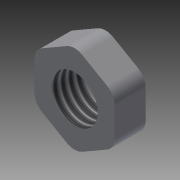
# Autodesk Inventor part: gaika3-2
Saved by Autodesk Inventor 2015 (Build 190159000, 159)
## iProperties
Created: 2016-05-20
Part Number: gaika3-2
Material: Generic
Document SubType Name: Modeling
Designer: Kostya
Density: 1 g/cm^3
Appearance: Default
Author: Kostya
Autodesk Inventor part; units mm, degrees
ref_plane "YZ Plane" through (0, 0, 0) normal (1, 0, 0) x (0, 1, 0)
ref_plane "XZ Plane" through (0, 0, 0) normal (0, 1, 0) x (-1, 0, 0)
ref_plane "XY Plane" through (0, 0, 0) normal (0, 0, 1) x (1, 0, 0)
sketch "Sketch1" plane through (0, 0, 0) normal (0, 1, 0) x (-1, 0, 0)
  line L0 (0.5, 2.7113) -> (2.0981, 1.7887)
  line L1 (2.5981, 0.9226) -> (2.5981, -0.9226)
  line L2 (2.0981, -1.7887) -> (0.5, -2.7113)
  line L3 (-0.5, -2.7113) -> (-2.0981, -1.7887)
  line L4 (-2.5981, -0.9226) -> (-2.5981, 0.9226)
  line L5 (-2.0981, 1.7887) -> (-0.5, 2.7113)
  circle A0 centre (0, 0) radius 1.5
  arc A1 (2.5981, 0.9226) -> (2.0981, 1.7887) centre (1.5981, 0.9226) ccw
  arc A2 (2.0981, -1.7887) -> (2.5981, -0.9226) centre (1.5981, -0.9226) ccw
  arc A3 (0.5, 2.7113) -> (-0.5, 2.7113) centre (0, 1.8453) ccw
  arc A4 (-2.0981, 1.7887) -> (-2.5981, 0.9226) centre (-1.5981, 0.9226) ccw
  arc A5 (-2.5981, -0.9226) -> (-2.0981, -1.7887) centre (-1.5981, -0.9226) ccw
  arc A6 (-0.5, -2.7113) -> (0.5, -2.7113) centre (0, -1.8453) ccw
  point P0 (0, 3)
  point P1 (2.5981, 1.5)
  point P2 (2.5981, -1.5)
  point P3 (0, -3)
  point P4 (-2.5981, -1.5)
  point P5 (-2.5981, 1.5)
  dimension "d0" = 6
  dimension "d1" = 3
  dimension "d2" = 1
  constraints: 12 end point, 12 point on circle, 12 point on line, 12 tangent, 7 centre point, 5 equal radius, 2 coincident, 13 other
  measures "d0" distance of point (0, -3) point (0, 3)
  measures "d1" diameter of A0
  measures "d2" radius of A1
extrude "Extrusion1" add sketch "Sketch1" along normal blind 2
thread "Thread1" size "M3x0.5" class "6H" standard "ANSI Metric M Profile" full length
body "Solid1"
